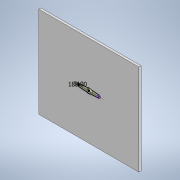
# Autodesk Inventor part: Base
Saved by Autodesk Inventor 2020 (Build 240168000, 168)
## iProperties
Created: 2020-02-28
Part Number: Base
Material: Generic
Document SubType Name: Modeling
Designer: othscs164
Density: 1 g/cm^3
Appearance: Default
Author: othscs164
Autodesk Inventor part; units mm, degrees
ref_plane "YZ Plane" through (0, 0, 0) normal (1, 0, 0) x (0, 1, 0)
ref_plane "XZ Plane" through (0, 0, 0) normal (0, 1, 0) x (-1, 0, 0)
ref_plane "XY Plane" through (0, 0, 0) normal (0, 0, 1) x (1, 0, 0)
sketch "Sketch2" plane through (0, 0, 0) normal (0, 0, 1) x (1, 0, 0)
  line L0 (-19.05, -12.7) -> (19.05, -12.7)
  line L1 (19.05, -12.7) -> (19.05, 12.7)
  line L2 (19.05, 12.7) -> (-19.05, 12.7)
  line L3 (-19.05, 12.7) -> (-19.05, -12.7)
  line L4 (-19.05, -12.7) -> (19.05, 12.7) construction
  line L5 (19.05, -12.7) -> (-19.05, 12.7) construction
  point P0 (0, 0)
  dimension "d0" = 38.1
  dimension "d1" = 25.4
  constraints: 12 end point, 2 midpoint, 2 parallel, 1 horizontal, 1 perpendicular
  measures "d0" distance of L2.end L1.end
  measures "d1" distance of L1.end L0.end
extrude "Extrusion1" add sketch "Sketch2" along normal blind 3.175
sketch "Sketch3" plane through (0, 0, 3.175) normal (0, 0, 1) x (1, 0, 0)
  line L0 (2.1333, -2.875) -> (14.1462, -1.9947)
  line L1 (14.1462, 1.9947) -> (2.1333, 2.875)
  line L2 (-2.1333, 2.875) -> (-14.1462, 1.9947)
  line L3 (-14.1462, -1.9947) -> (-2.1333, -2.875)
  arc A0 (2.1333, 2.875) -> (-2.1333, 2.875) centre (0, 0) ccw
  arc A1 (-2.1333, -2.875) -> (2.1333, -2.875) centre (0, 0) ccw
  arc A2 (14.1462, -1.9947) -> (14.1462, 1.9947) centre (14, 0) ccw
  arc A3 (-14.1462, 1.9947) -> (-14.1462, -1.9947) centre (-14, 0) ccw
  point P0 (0, 0)
  constraints: 8 end point, 8 point on circle, 4 centre point, 2 parallel, 1 tangent
extrude "Extrusion2" cut sketch "Sketch3" against normal blind 1.65
ref_plane "Work Plane1" through (-19.05, 0, 0) normal (0, -1, 0) x (1, 0, 0)
sketch "Sketch4" plane through (-19.05, 0, 0) normal (0, -1, 0) x (1, 0, 0)
  line L0 (3.05, 3.175) -> (4.9038, 3.175) projected
  line L1 (3.05, 3.175) -> (3.05, 1.525) projected
  line L2 (3.05, 3.175) -> (3.304, 2.6748)
  line L3 (3.304, 2.6748) -> (3.05, 2.6748)
  line L4 (3.304, 2.6748) -> (3.558, 2.6748) construction
  line L5 (3.05, 3.175) -> (3.05, 2.6748)
  line L6 (3.05, 3.175) -> (3.05, 1.525) projected
  point P0 (19.05, 0)
  dimension "d7" = 180
  dimension "d8" = 0.254
  constraints: 8 end point, 2 collinear, 1 horizontal, 1 point on line
  measures "d7" angle of L3 L4
  measures "d8" distance of L2.end L3.end
sketch "Sketch5" plane through (-19.05, 0, 0) normal (0, -1, 0) x (1, 0, 0)
  point P0 (19.05, 0)
sketch "Sketch6" plane through (19.05, -12.7, 0) normal (1, 0, 0) x (0, 0, -1)
  line L0 (0, 0) -> (0, 25.4) projected
  line L1 (0, 25.4) -> (-3.175, 25.4) projected
  line L2 (-3.175, 0) -> (-3.175, 25.4) projected
  line L3 (0, 0) -> (-3.175, 0) projected
  point P0 (0, 12.7)
extrude "Extrusion3" add sketch "Sketch6" along normal blind 50.8
sketch "Sketch7" plane through (-19.05, -12.7, 0) normal (-1, 0, 0) x (0, 0, 1)
  line L0 (0, 25.4) -> (0, 0) projected
  line L1 (0, 0) -> (3.175, 0) projected
  line L2 (3.175, 25.4) -> (3.175, 0) projected
  line L3 (0, 25.4) -> (3.175, 25.4) projected
  point P0 (0, 12.7)
extrude "Extrusion4" add sketch "Sketch7" along normal blind 50.8
sketch "Sketch8" plane through (69.85, 12.7, 3.175) normal (0, 1, 0) x (1, 0, 0)
  line L0 (-139.7, 3.175) -> (0, 3.175) projected
  line L1 (-139.7, 0) -> (-139.7, 3.175) projected
  line L2 (-139.7, 0) -> (0, 0) projected
  line L3 (0, 3.175) -> (0, 0) projected
  point P0 (-69.85, 3.175)
extrude "Extrusion5" add sketch "Sketch8" along normal blind 50.8
sketch "Sketch9" plane through (69.85, -12.7, 0) normal (0, -1, 0) x (1, 0, 0)
  line L0 (0, 0) -> (-139.7, 0) projected
  line L1 (0, 3.175) -> (0, 0) projected
  line L2 (0, 3.175) -> (-139.7, 3.175) projected
  line L3 (-139.7, 0) -> (-139.7, 3.175) projected
  point P0 (-69.85, 0)
extrude "Extrusion6" add sketch "Sketch9" along normal blind 50.8
sketch "Sketch10" plane through (0, 0, 3.175) normal (0, 0, 1) x (1, 0, 0)
  line L0 (-14.1462, 1.9947) -> (-2.1333, 2.875) projected
  arc A0 (2.1333, 2.875) -> (-2.1333, 2.875) centre (0, 0) ccw projected
  line L1 (2.1333, 2.875) -> (14.1462, 1.9947) projected
  arc A1 (14.1462, -1.9947) -> (14.1462, 1.9947) centre (14, 0) ccw projected
  line L2 (14.1462, -1.9947) -> (2.1333, -2.875) projected
  arc A2 (-2.1333, -2.875) -> (2.1333, -2.875) centre (0, 0) ccw projected
  line L3 (-2.1333, -2.875) -> (-14.1462, -1.9947) projected
  arc A3 (-14.1462, 1.9947) -> (-14.1462, -1.9947) centre (-14, 0) ccw projected
  line L4 (-2.1333, -2.875) -> (-14.1462, -1.9947)
  line L5 (-14.1462, 1.9947) -> (-2.1333, 2.875)
  line L6 (2.1333, -2.875) -> (14.1462, -1.9947)
  line L7 (14.1462, 1.9947) -> (2.1333, 2.875)
  arc A4 (-2.1333, -2.875) -> (2.1333, -2.875) centre (0, 0) ccw
  arc A5 (2.1333, 2.875) -> (-2.1333, 2.875) centre (0, 0) ccw
  arc A6 (-14.1462, 1.9947) -> (-14.1462, -1.9947) centre (-14, 0) ccw
  arc A7 (14.1462, -1.9947) -> (14.1462, 1.9947) centre (14, 0) ccw
  point P0 (0, 0)
  constraints: 9 point on circle, 8 end point, 4 centre point, 4 tangent, 2 equal length, 1 concentric
sketch "Sketch11" plane through (0, 0, 1.525) normal (0, 0, 1) x (1, 0, 0)
  circle A0 centre (0, 0) radius 3.58
  constraints: 1 centre point, 1 coincident
extrude "Extrusion7" cut sketch "Sketch11" against normal up to surface (1.525 mm away)
body "Solid1"
